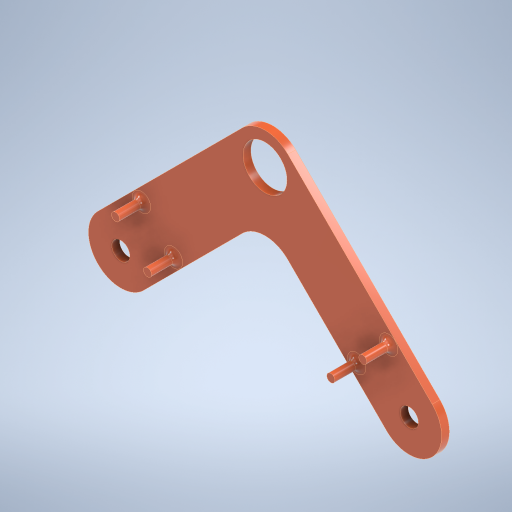
# Autodesk Inventor part: rockerbogieçükü
Saved by Autodesk Inventor 2023.2 (Build 272271000, 271)
## iProperties
Created: 2022-12-06
Part Number: rockerbogieçükü
Material: Generic
Document SubType Name: Modeling
Designer: omrfrkmll
Density: 1 g/cm^3
Appearance: Smooth - Light Orange
Author: omrfrkmll
Autodesk Inventor part; units mm, degrees
ref_plane "YZ Plane" through (0, 0, 0) normal (1, 0, 0) x (0, 1, 0)
ref_plane "XZ Plane" through (0, 0, 0) normal (0, 1, 0) x (-1, 0, 0)
ref_plane "XY Plane" through (0, 0, 0) normal (0, 0, 1) x (1, 0, 0)
sketch "Sketch1" plane through (0, 0, 0) normal (0, 0, 1) x (1, 0, 0)
  line L0 (0, 12.7112) -> (0, -15.7964)
  line L1 (-14.6857, 0) -> (16.9071, 0)
  line L2 (8.8388, 8.8388) -> (64.6598, -46.9822)
  line L3 (-8.8388, 8.8388) -> (-64.6598, -46.9822)
  line L4 (8.8388, -26.5165) -> (46.9822, -64.6598)
  line L5 (-8.8388, -26.5165) -> (-46.9822, -64.6598)
  arc A0 (8.8388, 8.8388) -> (-8.8388, 8.8388) centre (0, 0) ccw
  arc A1 (8.8388, -26.5165) -> (-8.8388, -26.5165) centre (0, -35.3553) ccw
  arc A2 (46.9822, -64.6598) -> (64.6598, -46.9822) centre (55.821, -55.821) ccw
  arc A3 (-64.6598, -46.9822) -> (-46.9822, -64.6598) centre (-55.821, -55.821) ccw
  circle A4 centre (-55.821, -55.821) radius 3.5
  circle A5 centre (55.821, -55.821) radius 3.5
  circle A6 centre (0, 0) radius 8.5
  point P0 (0, 17.6777)
  point P1 (0, -17.6777)
  dimension "d0" = 25
  dimension "d1" = 12.5
  dimension "d2" = 0
  dimension "d3" = 90
  dimension "d4" = 7
  dimension "d5" = 7
  dimension "d8" = 17
  dimension "d17" = 55.821
  constraints: 12 end point, 8 point on circle, 8 tangent, 7 centre point, 7 point on line, 3 coincident, 2 horizontal, 2 parallel, 2 vertical, 1 equal radius, 1 perpendicular, 3 other
  measures "d0" distance between parallel lines of L2 L4
  measures "d1" radius of A0
  measures "d2" distance of point (0, 0) A0.centre
  measures "d3" angle of L2 L3
  measures "d4" diameter of A4
  measures "d5" diameter of A5
  measures "d8" diameter of A6
  measures "d17" horizontal distance of A2.centre point (0, 0)
extrude "Extrusion1" add sketch "Sketch1" along normal blind 3
sketch "Sketch2" plane through (0, 0, 3) normal (0, 0, 1) x (1, 0, 0)
  circle A0 centre (55.821, -55.821) radius 3.5 projected
  line L0 (55.821, -55.821) -> (31.101, -31.101)
  line L1 (64.6598, -46.9822) -> (8.8388, 8.8388) projected
  circle A1 centre (47.8308, -35.4564) radius 1.55
  circle A2 centre (35.4564, -47.8308) radius 1.55
  point P0 (0, 0)
  dimension "d9" = 3.1
  dimension "d10" = 3.1
  dimension "d11" = 21.876
  dimension "d12" = 17.5
  constraints: 2 centre point, 2 end point, 1 parallel, 1 symmetric about line
  measures "d9" diameter of A1
  measures "d10" diameter of A2
  measures "d11" distance of L0.start A1.centre
  measures "d12" distance of A2.centre A1.centre
extrude "Extrusion2" add sketch "Sketch2" along normal blind 10 contours A1 | A2
mirror "Mirror1" about plane through (0, 0, 0) normal (1, 0, 0) of "Extrusion2"
fillet "Fillet1" radius 2 4 edges at (-46.2808, -35.4564, 3) (-33.9064, -47.8308, 3) (46.2808, -35.4564, 3) (33.9064, -47.8308, 3)
body "Solid1"
